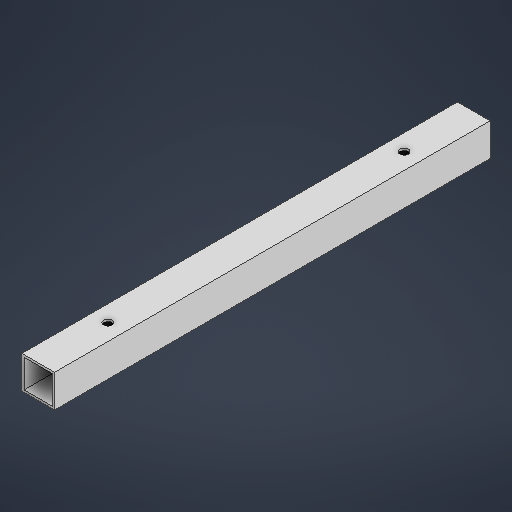
# Autodesk Inventor part: 15x152
Saved by Autodesk Inventor 2025 (Build 290162000, 162)
## iProperties
Created: 2025-04-22
Part Number: 15x152
Material: 常规
Document SubType Name: Modeling
Designer: XH
Density: 1 g/cm^3
Appearance: 默认
Author: XH
Autodesk Inventor part; units mm, degrees
ref_plane "YZ Plane" through (0, 0, 0) normal (1, 0, 0) x (0, 1, 0)
ref_plane "XZ Plane" through (0, 0, 0) normal (0, 1, 0) x (-1, 0, 0)
ref_plane "XY Plane" through (0, 0, 0) normal (0, 0, 1) x (1, 0, 0)
sketch "草图1" plane through (0, 0, 0) normal (0, 0, 1) x (1, 0, 0)
  line L0 (7.5, -7.5) -> (-7.5, -7.5)
  line L1 (-7.5, -7.5) -> (-7.5, 7.5)
  line L2 (-7.5, 7.5) -> (7.5, 7.5)
  line L3 (7.5, 7.5) -> (7.5, -7.5)
  line L4 (7.5, -7.5) -> (-7.5, 7.5) construction
  line L5 (-7.5, -7.5) -> (7.5, 7.5) construction
  line L6 (6.5, 6.5) -> (-6.5, 6.5)
  line L7 (-6.5, 6.5) -> (-6.5, -6.5)
  line L8 (-6.5, -6.5) -> (6.5, -6.5)
  line L9 (6.5, -6.5) -> (6.5, 6.5)
  point P0 (0, 0)
  dimension "d0" = 15
  dimension "d1" = 15
  dimension "d2" = 1
  constraints: 20 end point, 4 parallel, 2 midpoint, 2 perpendicular, 1 horizontal, 3 other
  measures "d0" distance of L1.end L2.end
  measures "d1" distance of L2.end L0.start
  measures "d2" distance between parallel lines of L2 L6
extrude "拉伸1" add sketch "草图1" along normal blind 200
sketch "草图2" plane through (-7.5, -7.5, 0) normal (0, -1, 0) x (1, 0, 0)
  line L0 (14, 200) -> (1, 200) projected
  line L1 (7.5, 200) -> (7.5, 0)
  line L2 (7.5, 100) -> (64.493, 100)
  circle A0 centre (7.5, 168) radius 2
  circle A1 centre (7.5, 32) radius 2
  dimension "d5" = 4
  dimension "d8" = 68
  constraints: 4 end point, 2 centre point, 2 midpoint, 1 horizontal, 1 point on line, 1 symmetric about line, 1 vertical, 1 other
  measures "d5" diameter of A0
  measures "d8" distance from line of A1.centre L2
extrude "拉伸2" cut sketch "草图2" against normal blind 300
